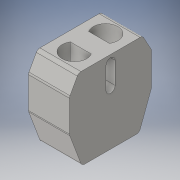
# Autodesk Inventor part: Nathan_Sensor_Motor
Saved by Autodesk Inventor 2016 (Build 200138000, 138)
## iProperties
Created: 2016-12-12
Part Number: Nathan_Sensor_Motor
Material: Generic
Document SubType Name: Modeling
Designer: Student
Density: 1 g/cm^3
Appearance: Default
Author: Student
Autodesk Inventor part; units mm, degrees
ref_plane "YZ Plane" through (0, 0, 0) normal (1, 0, 0) x (0, 1, 0)
ref_plane "XZ Plane" through (0, 0, 0) normal (0, 1, 0) x (-1, 0, 0)
sketch "Sketch1" plane through (0, 0, 0) normal (1, 0, 0) x (0, 1, 0)
  line L0 (0, 0) -> (-25.4, 0)
  line L1 (-25.4, 0) -> (-25.4, 25.4)
  line L2 (-25.4, 25.4) -> (0, 25.4)
  line L3 (0, 25.4) -> (0, 0)
  dimension "d0" = 25.4
  dimension "d1" = 25.4
  constraints: 8 end point, 2 parallel, 1 horizontal, 1 perpendicular
  measures "d0" distance of L1.end L2.end
  measures "d1" distance of L0.end L1.end
extrude "Extrusion1" add sketch "Sketch1" along normal blind 12.7
sketch "Sketch2" plane through (0, 0, 25.4) normal (0, 1, 0) x (1, 0, 0)
  line L0 (0, 0) -> (0, 25.4) projected
  line L1 (0, 12.7) -> (12.7, 12.7)
  line L2 (12.7, 25.4) -> (12.7, 0) projected
  line L3 (0, 11.684) -> (0, 12.7)
  line L4 (0, 12.7) -> (0, 13.716)
  dimension "d4" = 1.016
  dimension "d5" = 1.016
  constraints: 6 end point, 2 midpoint, 2 point on line, 1 collinear
  measures "d4" distance of L3.start L1.start
  measures "d5" distance of L4.end L1.start
ref_plane "Work Plane1" through (6.35, 0, 25.4) normal (1, 0, 0) x (0, 0, -1)
sketch "Sketch3" plane through (6.35, 0, 25.4) normal (1, 0, 0) x (0, 0, -1)
  line L0 (13.7199, 0.3391) -> (13.7199, -24.4131)
  line L1 (13.7199, 0.3391) -> (21.3333, 0.3391)
  line L2 (17.5266, 0.3391) -> (17.5266, -24.4131)
  line L3 (21.3333, 0.3391) -> (21.3333, -24.4131)
  line L4 (21.3333, -24.4131) -> (13.7199, -24.4131)
  point P0 (25.4, 0)
  point P1 (17.5266, -26.1924)
  constraints: 10 end point, 2 midpoint, 1 horizontal, 1 perpendicular, 1 vertical
revolve "Revolution1" cut sketch "Sketch3" angle 360 about axis through (6.35, 0.3391, 7.8734) along (0, -1, 0) contours L1 L3 L4 L2
sketch "Sketch4" plane through (6.35, 0, 25.4) normal (1, 0, 0) x (0, 0, -1)
  line L0 (11.6726, 0.4635) -> (11.6726, -24.4067)
  line L1 (0, -25.4) -> (25.4, -25.4) projected
  line L2 (11.6726, 0.4635) -> (4.0526, 0.4635)
  line L3 (4.0526, 0.4635) -> (4.1052, 0)
  line L4 (7.8626, 0.4635) -> (7.8626, -24.4067)
  line L5 (4.0526, -24.4067) -> (4.0526, 0.4635)
  line L6 (25.4, 0) -> (0, 0) projected
  line L7 (4.0789, 0) -> (4.0526, 0.4635)
  line L8 (11.6726, -24.4067) -> (4.0526, -24.4067)
  point P0 (7.1058, -26.4153)
  dimension "d7" = 7.62
  constraints: 14 end point, 3 perpendicular, 3 point on line, 2 midpoint, 1 horizontal
  measures "d7" distance of L0.start L2.end
revolve "Revolution2" cut sketch "Sketch4" angle 360 about axis through (6.35, 0.4635, 17.5374) along (0, -1, 0) contours L4 L6 L3 L2 | L4 L8 L5 L6 | L7 L6 L5 | L3 L6 L7
sketch "Sketch5" plane through (0, 0, 0) normal (-1, 0, 0) x (0, 0, 1)
  line L0 (0, 0) -> (0, -25.4) projected
  line L1 (0, -25.4) -> (3.81, -25.4)
  line L2 (0, -25.4) -> (25.4, -25.4) projected
  line L3 (0, -25.4) -> (0, 0) projected
  line L4 (0, -25.4) -> (0, -15.24)
  line L5 (0, -15.24) -> (3.81, -25.4)
  dimension "d9" = 3.81
  dimension "d10" = 10.16
  constraints: 6 end point, 2 point on line
  measures "d9" distance of L0.end L1.end
  measures "d10" distance of L0.end L4.end
extrude "Extrusion2" cut sketch "Sketch5" against normal blind 12.7
sketch "Sketch6" plane through (0, 0, 0) normal (-1, 0, 0) x (0, 0, 1)
  line L0 (25.4, -25.4) -> (3.81, -25.4) projected
  line L1 (25.4, -25.4) -> (21.59, -25.4)
  line L2 (25.4, -25.4) -> (25.4, -15.24)
  line L3 (25.4, 0) -> (25.4, -25.4) projected
  line L4 (25.4, -15.24) -> (21.59, -25.4)
  point P0 (0, 0)
  dimension "d13" = 3.81
  dimension "d14" = 10.16
  constraints: 6 end point, 2 point on line
  measures "d13" distance of L0.start L1.end
  measures "d14" distance of L0.start L2.end
extrude "Extrusion3" cut sketch "Sketch6" against normal blind 12.7
sketch "Sketch7" plane through (0, 0, 0) normal (-1, 0, 0) x (0, 0, 1)
  line L0 (25.4, 0) -> (22.606, 0)
  line L1 (25.4, 0) -> (0, 0) projected
  line L2 (25.4, 0) -> (25.4, -5.08)
  line L3 (25.4, -15.24) -> (25.4, 0) projected
  line L4 (25.4, -5.08) -> (22.606, 0)
  dimension "d17" = 2.794
  dimension "d18" = 5.08
  constraints: 6 end point, 2 point on line
  measures "d17" distance of L0.start L0.end
  measures "d18" distance of L0.start L2.end
extrude "Extrusion4" cut sketch "Sketch7" against normal blind 12.7
sketch "Sketch8" plane through (0, 0, 0) normal (-1, 0, 0) x (0, 0, 1)
  line L0 (0, 0) -> (2.794, 0)
  line L1 (0, 0) -> (22.606, 0) projected
  line L2 (0, 0) -> (0, -5.08)
  line L3 (0, 0) -> (0, -15.24) projected
  line L4 (0, -5.08) -> (2.794, 0)
  dimension "d21" = 2.794
  dimension "d22" = 5.08
  constraints: 6 end point, 2 point on line
  measures "d21" distance of L0.start L0.end
  measures "d22" distance of L0.start L2.end
extrude "Extrusion5" cut sketch "Sketch8" against normal blind 12.7
sketch "Sketch9" plane through (0, -25.4, 3.81) normal (0, -1, 0) x (1, 0, 0)
  circle A0 centre (6.35, 4.0634) radius 3.8067 projected
  line L0 (6.35, 7.8701) -> (6.35, 7.856)
  circle A1 centre (6.35, 5.5721) radius 2.2839
  point P0 (0, -3.81)
  constraints: 2 end point, 2 vertical alignment, 1 vertical, 3 other
extrude "Extrusion6" cut sketch "Sketch9" along normal mid plane 12.7 contours A1
sketch "Sketch10" plane through (0, -25.4, 3.81) normal (0, -1, 0) x (1, 0, 0)
  line L0 (0, 18.796) -> (0, -1.016) projected
  circle A0 centre (6.3413, 12.1953) radius 2.286
  point P0 (0, -3.81)
  constraints: 1 centre point
extrude "Extrusion7" cut sketch "Sketch10" along normal mid plane 12.7
sketch "Sketch11" plane through (0, 0, 22.606) normal (0, 1, 0) x (1, 0, 0)
  line L0 (12.7, 19.812) -> (12.7, 0) projected
  line L1 (0, 0) -> (0, 19.812) projected
  line L2 (12.7, 12.6934) -> (0, 12.6934)
  line L3 (0, 12.6934) -> (0, 7.0597)
  line L4 (0, 7.0597) -> (12.7, 7.0597)
  line L5 (12.7, 7.0597) -> (12.7, 12.6934)
  point P0 (0, 22.606)
  constraints: 8 end point, 2 parallel, 2 point on line, 1 horizontal, 1 perpendicular
extrude "Extrusion8" add sketch "Sketch11" against normal blind 12.7
sketch "Sketch12" plane through (0, 0, 0) normal (-1, 0, 0) x (0, 0, 1)
  line L0 (2.794, 0) -> (22.606, 0) projected
  line L1 (12.7, 0) -> (12.7, -2.2773)
  arc A0 (14.1224, -2.2773) -> (11.2776, -2.2773) centre (12.7, -2.2773) ccw
  line L2 (11.2776, -2.2773) -> (11.2776, -8.998)
  arc A1 (11.2776, -8.998) -> (14.1224, -8.998) centre (12.7, -8.998) ccw
  line L3 (14.1224, -2.2773) -> (14.1224, -8.998)
  point P0 (0, 0)
  point P1 (12.7, -6.9532)
  dimension "d32" = 2.8448
  constraints: 6 end point, 4 point on circle, 3 vertical, 2 centre point, 1 coincident, 1 midpoint, 1 point on line, 1 tangent
  measures "d32" diameter of A0
extrude "Extrusion9" cut sketch "Sketch12" against normal blind 25.4
fillet "Fillet1" radius 1.27 8 edges at (6.35, 0, 2.794) (6.35, -5.08, 0) (6.35, -15.24, 0) (6.35, -25.4, 3.81) (6.35, 0, 22.606) (6.35, -5.08, 25.4) (6.35, -15.24, 25.4) (6.35, -25.4, 21.59)
body "Solid1"
